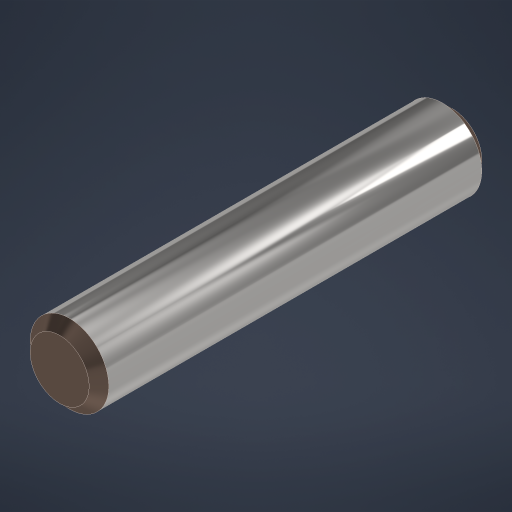
# Autodesk Inventor part: Pin
Saved by Autodesk Inventor 2023 (Build 270158000, 158)
## iProperties
Created: 2022-11-29
Part Number: Pin
Material: Steel
Document SubType Name: Modeling
Designer: iusti
Density: 7.85 g/cm^3
Appearance: Gunmetal - Antique Polished
Author: iusti
Autodesk Inventor part; units mm, degrees
ref_plane "YZ Plane" through (0, 0, 0) normal (1, 0, 0) x (0, 1, 0)
ref_plane "XZ Plane" through (0, 0, 0) normal (0, 1, 0) x (-1, 0, 0)
ref_plane "XY Plane" through (0, 0, 0) normal (0, 0, 1) x (1, 0, 0)
sketch "Sketch1" plane through (0, 0, 0) normal (1, 0, 0) x (0, 1, 0)
  line L0 (2, 10) -> (0, 10)
  line L1 (0, 10) -> (0, -10)
  line L2 (0, -10) -> (2, -10)
  line L3 (2, -10) -> (2, 10)
  point P0 (0, 0)
  point P1 (0, 0)
  dimension "d0" = 4
  dimension "d1" = 20
  constraints: 8 end point, 2 parallel, 1 coincident, 1 horizontal, 1 midpoint, 1 perpendicular
  measures "d0" diameter of L3 L1
  measures "d1" distance of L2.end L0.start
revolve "Revolution1" add sketch "Sketch1" angle 360 about axis through (0, 0, 10) along (0, 0, -1)
chamfer "Chamfer1" distance 0.5 angle 45 2 edges at (0, -2, 10) (0, -2, -10)
body "Solid1"
